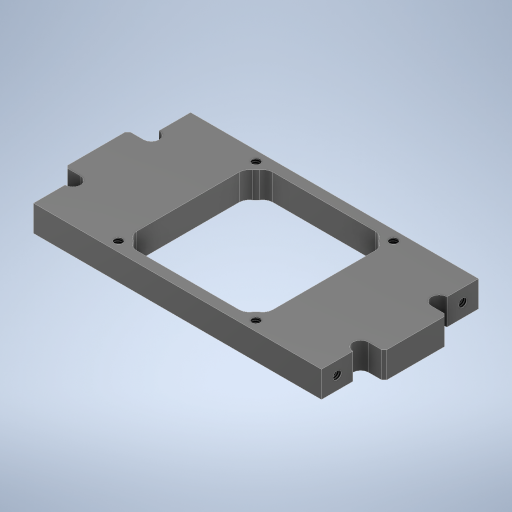
# Autodesk Inventor part: HeadCameraMountFrame
Saved by Autodesk Inventor 2024.2 (Build 282272000, 272)
## iProperties
Created: 2024-01-19
Part Number: HeadCameraMountFrame
Material: Acetal Resin, Black
Document SubType Name: Modeling
Designer: Masato Kubotera
Density: 1.425 g/cm^3
Appearance: Smooth - Black
Mass: 7.65641 g
Surface Area: 38.5811 cm^2
Volume: 5.37292 cm^3
Vendor: meviy
Author: Masato Kubotera
Autodesk Inventor part; units mm, degrees
ref_plane "YZ Plane" through (0, 0, 0) normal (1, 0, 0) x (0, 1, 0)
ref_plane "XZ Plane" through (0, 0, 0) normal (0, 1, 0) x (-1, 0, 0)
ref_plane "XY Plane" through (0, 0, 0) normal (0, 0, 1) x (1, 0, 0)
sketch "Sketch1" plane through (0, 0, 0) normal (0, 0, 1) x (1, 0, 0)
  line L0 (15, 27.5) -> (-15, 27.5)
  line L1 (-15, 27.5) -> (-15, -27.5)
  line L2 (-15, -27.5) -> (15, -27.5)
  line L3 (15, -27.5) -> (15, 27.5)
  line L4 (15, 27.5) -> (-15, -27.5) construction
  line L5 (-15, 27.5) -> (15, -27.5) construction
  line L6 (13.14, 13.14) -> (-13.14, 13.14) construction
  line L7 (-13.14, 13.14) -> (-13.14, -13.14) construction
  line L8 (-13.14, -13.14) -> (13.14, -13.14) construction
  line L9 (13.14, -13.14) -> (13.14, 13.14) construction
  line L10 (13.14, 13.14) -> (-13.14, -13.14) construction
  line L11 (-13.14, 13.14) -> (13.14, -13.14) construction
  line L12 (15, 15) -> (-15, 15) construction
  line L13 (-15, 15) -> (-15, -15) construction
  line L14 (-15, -15) -> (15, -15) construction
  line L15 (15, -15) -> (15, 15) construction
  line L16 (15, 15) -> (-15, -15) construction
  line L17 (-15, 15) -> (15, -15) construction
  line L18 (0, 27.5) -> (0, -27.5) construction
  line L19 (15, 0) -> (-15, 0) construction
  line L20 (6, 27.5) -> (6, 30.5)
  line L21 (6, 30.5) -> (-6, 30.5)
  line L22 (-6, 30.5) -> (-6, 27.5)
  arc A0 (-9, 27.5) -> (-6, 27.5) centre (-7.5, 27.5) ccw
  arc A1 (11.1449, 13) -> (13, 11.1449) centre (13.14, 13.14) ccw
  line L23 (-15.1, -15.1) -> (15.1, 15.1) construction
  line L24 (15.1, -15.1) -> (-15.1, 15.1) construction
  line L25 (6, -27.5) -> (6, -30.5)
  line L26 (6, -30.5) -> (-6, -30.5)
  line L27 (-6, -30.5) -> (-6, -27.5)
  arc A2 (-6, -27.5) -> (-9, -27.5) centre (-7.5, -27.5) ccw
  line L28 (-12, 27.5) -> (-12, 21.5) construction
  line L29 (0, 30.5) -> (0, 27.5) construction
  line L30 (12, 27.5) -> (12, 21.5) construction
  arc A3 (6, 27.5) -> (9, 27.5) centre (7.5, 27.5) ccw
  line L31 (12, -27.5) -> (12, -21.5) construction
  arc A4 (9, -27.5) -> (6, -27.5) centre (7.5, -27.5) ccw
  arc A5 (13, -11.1449) -> (11.1449, -13) centre (13.14, -13.14) ccw
  arc A6 (-13, 11.1449) -> (-11.1449, 13) centre (-13.14, 13.14) ccw
  arc A7 (-11.1449, -13) -> (-13, -11.1449) centre (-13.14, -13.14) ccw
  line L32 (13, -11.1449) -> (13, 11.1449)
  line L33 (11.1449, 13) -> (-11.1449, 13)
  line L34 (-13, 11.1449) -> (-13, -11.1449)
  line L35 (-11.1449, -13) -> (11.1449, -13)
  point P0 (0, 0)
  point P1 (0, 0)
  point P2 (0, 0)
  point P3 (13.14, -13.14)
  point P4 (-9, -27.5)
  point P5 (6, 28)
  point P6 (6, -27.5)
  point P7 (-6, -27.5)
  point P8 (-6, -27.5)
  point P9 (6, -27.5)
  point P10 (9, -27.5)
  dimension "d0" = 26.28
  dimension "d1" = 26.28
  dimension "d2" = 30
  dimension "d3" = 30
  dimension "d19" = 3
  dimension "d20" = 12
  dimension "d26" = 2
  dimension "d37" = 55
  dimension "d40" = 6
  dimension "d41" = 6
  dimension "d50" = 12.5
  dimension "d57" = 30
  dimension "d60" = 1.5
  dimension "d61" = 2
  constraints: 70 end point, 23 symmetric about line, 16 midpoint, 16 point on circle, 9 parallel, 8 centre point, 5 vertical, 4 coincident, 4 horizontal, 3 point on line, 2 perpendicular, 1 collinear, 1 tangent, 17 other
  measures "d0" distance of L8.end L7.end
  measures "d1" distance of L7.end L6.end
  measures "d2" distance of L14.end L13.end
  measures "d3" distance of L13.end L12.end
  measures "d19" distance of L20.start L20.end
  measures "d20" distance of L20.end L21.end
  measures "d26" radius of A1
  measures "d37" distance of L2.end L3.end
  measures "d40" distance of L28.start L28.end
  measures "d41" distance between parallel lines of L22 L28
  measures "d50" distance between parallel lines of L14 L2
  measures "d57" distance between parallel lines of L1 L3
  measures "d60" radius of A3
  measures "d61" distance between parallel lines of L3 L32
extrude "Extrusion1" add sketch "Sketch1" against normal blind 5 contours L3 L2 A4 A2 L1 L0 A0 A3 | L0 L22 L21 L20 | L25 L26 L27 L2 | A1 L32 A5 L35 A7 L34 A6 L33
hole "Hole1" at (13.14, 13.14, 0) at (-13.14, 13.14, 0) at (-13.14, -13.14, 0) at (13.14, -13.14, 0) direction (0, 0, -1) diameter 1.567 end through all thread size "M2x0.4" class "6H" standard "ANSI Metric M Profile"
extrude "Extrusion2" cut sketch "Sketch1" against normal through all contours A1 L32 A5 L35 A7 L34 A6 L33
sketch "Sketch2" plane through (-15, 27.5, 0) normal (0, 1, 0) x (1, 0, 0)
  line L0 (3, 5) -> (3, 0)
  line L1 (30, 0) -> (0, 0) projected
  line L2 (27, 5) -> (27, 0)
  line L3 (24, 5) -> (30, 5) projected
  line L4 (0, 5) -> (6, 5) projected
  point P0 (15, 0)
  point P1 (6, 0)
  point P2 (3, 2.5)
  point P3 (3, 0)
  point P4 (27, 2.5)
  point P5 (27, 0)
  constraints: 4 end point, 4 midpoint, 2 vertical, 1 other
hole "Hole2" at (-12, 27.5, -2.5) at (12, 27.5, -2.5) direction (0, -1, 0) diameter 1.567 depth 6.3 thread size "M2x0.4" class "6H" standard "ANSI Metric M Profile"
mirror "Mirror1" about plane through (0, 0, 0) normal (0, 1, 0) of "Hole2"
chamfer "Chamfer1" distance 0.5 angle 45 4 edges at (6, -30.5, -2.5) (-6, -30.5, -2.5) (6, 30.5, -2.5) (-6, 30.5, -2.5)
fillet "Fillet1" radius 2 8 edges at (13, 11.1449, -2.5) (11.1449, 13, -2.5) (13, -11.1449, -2.5) (11.1449, -13, -2.5) (-11.1449, -13, -2.5) (-13, -11.1449, -2.5) (-11.1449, 13, -2.5) (-13, 11.1449, -2.5)
body "Solid1"
